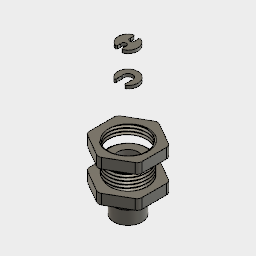
connector_bulkheads (Autodesk Fusion 360 design; units mm, degrees)
Autodesk Fusion 360 part; units mm, degrees
sketch "main sketch for revolve" plane through (0, 0, 0) normal (0, 0, 1) x (1, 0, 0)
  line L0 (0, 0) -> (0, 65) construction
  line L1 (10, 0) -> (10, 25)
  line L2 (10, 25) -> (20, 25)
  line L3 (20, 25) -> (20, 10)
  line L4 (20, 10) -> (30, 10)
  line L5 (10, 0) -> (30, 0)
  line L6 (30, 0) -> (30, 10)
  line L7 (30, 30.7607) -> (20, 30.7607)
  line L8 (20, 30.7607) -> (20, 40.7607)
  line L9 (20, 40.7607) -> (30, 40.7607)
  line L10 (30, 40.7607) -> (30, 30.7607)
  line L11 (10, 0) -> (10, -23.0706)
  line L12 (10, -23.0706) -> (14, -23.0706)
  line L13 (14, -23.0706) -> (14.6041, 0)
  dimension "d1" = 10
  dimension "d2" = 10
  dimension "d3" = 10
  dimension "d4" = 10
  dimension "d5" = 15
  dimension "d7" = 10
  dimension "d12" = 1.5
  dimension "d13" = 14
  constraint coincident L0.start origin
  constraint vertical L0
  constraint vertical L1
  constraint perpendicular L1 L2
  constraint perpendicular L2 L3
  constraint perpendicular L1 L4
  constraint perpendicular L1 L5
  constraint perpendicular L4 L6
  constraint horizontal L0.start origin
  constraint horizontal L7
  constraint vertical L8
  constraint horizontal L9
  constraint vertical L10
  constraint vertical L0.start
  constraint perpendicular L5 L11
  constraint perpendicular L11 L12
  constraint coincident L5
  measures "d1" distance of L0.start
  measures "d2" distance of L0 L1
  measures "d4" distance of L1 L3
  measures "d7" distance of L0.start
  measures "d12" angle of L11 L13
revolve "Revolve1" add sketch "main sketch for revolve" angle 360 about axis through (0, 0, 0) along (0, 1, 0) contours L1 L2 L3 L4 L5 L6 | L5 L11 L12 L13 makes body 1
thread "Thread1" "ISO Metric profile 39.0 M39x3 6g" major diameter 38.7645 minor diameter 35.3299 pitch 3 angle 60 modelled right hand crest width 0.375 on face at (19.9751, 20, 0.9969) crest through (19.3822, 25.1875, 0) on bodies 1
revolve "Revolve2" add sketch "main sketch for revolve" angle 360 about axis through (0, 0, 0) along (0, 1, 0) separate body contours L7 L8 L9 L10 makes body 2
thread "Thread2" "ISO Metric profile 40.0 M40x3 6H" major diameter 40.349 minor diameter 37.0024 pitch 3 angle 60 modelled right hand crest width 0.375 on face at (19.9751, 34.094, 0.9969) crest through (18.5012, 42.4482, 0) on bodies 2
sketch "make hex" plane through (0, 40.7607, 0) normal (0, 1, 0) x (-1, 0, 0)
  spline S0 degree 3 poles (-8.8216, 18.1436) (-6.4347, 19.1855) (-3.8685, 19.7549) (1.2964, 19.8694) (3.8449, 19.4292) (8.5883, 17.6042) (10.7431, 16.2519) (14.3776, 12.8203) (15.833, 10.7856) (17.4597, 7.1881) (17.9068, 5.7823) (18.4593, 2.9097) (18.5662, 1.4536) (18.5012, 0) knots 0 0 0 0 0.781349 0.781349 1.550392 1.550392 2.307125 2.307125 3.051545 3.051545 3.493239 3.493239 3.930425 3.930425 3.930425 3.930425
  arc A0 (13.0823, -13.0823) -> (18.5012, 0) centre (0, 0) ccw
  spline S1 degree 3 poles (13.0823, -13.0823) (11.4443, -14.8736) (9.4698, -16.3248) (5.0403, -18.4137) (2.6216, -19.0169) (-2.353, -19.2721) (-4.8615, -18.9058) (-9.6395, -17.2256) (-11.8576, -15.913) (-14.9269, -13.1796) (-15.9628, -12.0112) (-17.7506, -9.4451) (-18.4935, -8.0544) (-19.0673, -6.5916) knots 0 0 0 0 0.728177 0.728177 1.468651 1.468651 2.221417 2.221417 2.986471 2.986471 3.452631 3.452631 3.92329 3.92329 3.92329 3.92329
  arc A1 (-8.8216, 18.1436) -> (-19.0673, -6.5916) centre (0, 0) ccw
  circle A2 centre (0, 0) radius 30
  circle A3 centre (0, 0) radius 40.0088
  line L0 (25.9808, -15) -> (25.9808, 15)
  line L1 (25.9808, 15) -> (0, 30)
  line L2 (0, 30) -> (-25.9808, 15)
  line L3 (-25.9808, 15) -> (-25.9808, -15)
  line L4 (-25.9808, -15) -> (0, -30)
  line L5 (0, -30) -> (25.9808, -15)
  circle A4 centre (0, 0) radius 26.0763 construction
  dimension "d15" = 52.1527
  constraint coincident A0.centre A1.centre
  constraint coincident A2 A0.centre
  constraint vertical L0
  measures "d15" diameter of A4
extrude "Extrude1" cut sketch "make hex" against normal through all contours A2 L0 | A2 L1 | A2 L5 | A2 L2 | A2 L4 | A2 L3 | A3 bodies 1 2
fillet "Fillet1" radius 5 12 edges at (0, 5, -30) (25.9808, 5, 15) (25.9808, 5, -15) (-25.9808, 5, -15) (-25.9808, 5, 15) (0, 5, 30) (0, 35.7607, -30) (25.9808, 35.7607, -15) (25.9808, 35.7607, 15) (-25.9808, 35.7607, -15) (-25.9808, 35.7607, 15) (0, 35.7607, 30) on bodies 1 2
fillet "Fillet2" radius 10 1 edges at (-13.6158, 0, -5.2811) on bodies 1
ref_plane "WorkPlane1" through (0, 90.7607, 0) normal (0, 1, 0) x (-1, 0, 0)
ref_plane "WorkPlane2" through (0, 120.7607, 0) normal (0, 1, 0) x (-1, 0, 0)
sketch "power_cable_centering_orig_sketch" plane through (0, 90.7607, 0) normal (0, 1, 0) x (1, 0, 0)
  circle A0 centre (0, 0) radius 10 construction
  line L0 (4.25, -1.479) -> (4.25, -14.1244)
  line L1 (-4.25, -1.479) -> (-4.25, -14.1244)
  arc A1 (2.8333, -9.5902) -> (-2.8333, -9.5902) centre (0, 0) ccw
  arc A2 (4.25, -1.479) -> (-4.25, -1.479) centre (0, 0) ccw
  line L2 (0, 0) -> (0, -6.5785) construction
  arc A3 (4.25, -14.1244) -> (-4.25, -14.1244) centre (0, 0) ccw
  dimension "d18" = 4.5
  dimension "d19" = 8.5
  dimension "d33" = 14.75
  constraint concentric A0 A2
  constraint coincident A0
  constraint vertical L0
  constraint parallel L0 L1
  constraint coincident A0.centre A1.centre
  constraint parallel L1 L2
  constraint horizontal A0.centre A1.centre
  measures "d18" radius of A2
  measures "d19" distance of L0 L1
  measures "d33" radius of A3
extrude "Extrude2" add sketch "power_cable_centering_orig_sketch" along normal blind 3 separate body contours L0 L1 A1 A2 makes body 3
fillet "Fillet3" radius 1 4 edges at (-4.25, 92.2607, 1.479) (4.25, 92.2607, 1.479) (-4.25, 92.2607, 9.0519) (4.25, 92.2607, 9.0519) on bodies 3
sketch "usb_centering_orig_sketch" plane through (0, 120.7607, 0) normal (0, 1, 0) x (1, 0, 0)
  circle A0 centre (0, 0) radius 10
  line L0 (-2.25, 4.6782) -> (-2.25, 9.4868)
  line L1 (2.25, 4.6782) -> (2.25, 9.4868)
  line L2 (2.25, -4.6782) -> (2.25, -9.4868)
  line L3 (-2.25, -4.6782) -> (-2.25, -9.4868)
  line L4 (0, -4) -> (0, 4) construction
  arc A1 (2.25, -4.6782) -> (-2.25, -4.6782) centre (0, -4) ccw
  arc A2 (-2.25, 4.6782) -> (2.25, 4.6782) centre (0, 4) ccw
  circle A3 centre (0, 0) radius 9.75
  dimension "d23" = 4.7
  dimension "d24" = 8
  dimension "d25" = 4.5
  dimension "d29" = 19.5
  constraint equal A1 A2
  constraint vertical A0.centre A3.centre
  constraint vertical L0
  constraint parallel L0 L1
  constraint parallel L1 L2
  constraint vertical L3
  constraint vertical A0.centre
  constraint coincident A0.centre A3.centre
  constraint midpoint A0.centre L4
  constraint coincident A3 A0.centre
  measures "d23" diameter of A2
  measures "d25" distance of L0 L1
  measures "d29" diameter of A3
extrude "Extrude3" add sketch "usb_centering_orig_sketch" along normal blind 3 separate body contours L0 L1 L2 L3 A1 A2 A3 makes body 4
fillet "Fillet4" radius 1 8 edges at (-2.25, 122.2607, 4.6782) (2.25, 122.2607, 4.6782) (2.25, 122.2607, -4.6782) (-2.25, 122.2607, -4.6782) (2.25, 122.2607, 9.4868) (-2.25, 122.2607, 9.4868) (-2.25, 122.2607, -9.4868) (2.25, 122.2607, -9.4868) on bodies 4
ref_plane "WorkPlane3" through (0, 123.7607, 0) normal (0, 1, 0) x (1, 0, 0)
sketch "usb centering dxf" plane through (0, 123.7607, 0) normal (0, 1, 0) x (1, 0, 0)
  arc A0 (3.6214, 9.0525) -> (2.25, 8.124) centre (3.25, 8.124) ccw
  line L0 (2.25, 8.124) -> (2.25, 4.8124)
  arc A1 (2.25, 4.8124) -> (2.2799, 4.5699) centre (3.25, 4.8124) ccw
  arc A2 (-2.2799, 4.5699) -> (2.2799, 4.5699) centre (0, 4) ccw
  arc A3 (-2.2799, 4.5699) -> (-2.25, 4.8124) centre (-3.25, 4.8124) ccw
  line L1 (-2.25, 4.8124) -> (-2.25, 8.124)
  arc A4 (-2.25, 8.124) -> (-3.6214, 9.0525) centre (-3.25, 8.124) ccw
  arc A5 (-3.6214, 9.0525) -> (-3.6214, -9.0525) centre (0, 0) ccw
  arc A6 (-3.6214, -9.0525) -> (-2.25, -8.124) centre (-3.25, -8.124) ccw
  line L2 (-2.25, -8.124) -> (-2.25, -4.8124)
  arc A7 (-2.25, -4.8124) -> (-2.2799, -4.5699) centre (-3.25, -4.8124) ccw
  arc A8 (2.2799, -4.5699) -> (-2.2799, -4.5699) centre (0, -4) ccw
  arc A9 (2.2799, -4.5699) -> (2.25, -4.8124) centre (3.25, -4.8124) ccw
  line L3 (2.25, -4.8124) -> (2.25, -8.124)
  arc A10 (2.25, -8.124) -> (3.6214, -9.0525) centre (3.25, -8.124) ccw
  arc A11 (3.6214, -9.0525) -> (3.6214, 9.0525) centre (0, 0) ccw
ref_plane "WorkPlane4" through (0, 93.7607, -0.474) normal (0, 1, 0) x (1, 0, 0)
sketch "power cable centering dxf" plane through (0, 93.7607, -0.4476) normal (0, 1, 0) x (1, 0, 0)
  arc A0 (4.2955, -1.7889) -> (4.25, -2.087) centre (5.25, -2.087) ccw
  line L0 (4.25, -2.087) -> (4.25, -7.7577)
  line L1 (-4.25, -7.7577) -> (-4.25, -2.087)
  arc A1 (-4.25, -2.087) -> (-4.2955, -1.7889) centre (-5.25, -2.087) ccw
  arc A2 (4.2955, -1.7889) -> (-4.2955, -1.7889) centre (0, -0.4476) ccw
  arc A3 (5.8333, -8.5699) -> (-5.8333, -8.5699) centre (0, -0.4476) ccw
  arc A4 (4.25, -7.7577) -> (5.8333, -8.5699) centre (5.25, -7.7577) ccw
  arc A5 (-5.8333, -8.5699) -> (-4.25, -7.7577) centre (-5.25, -7.7577) ccw
equation "d33 = ( ( 29.5 / 2 ) * 1 mm )"
